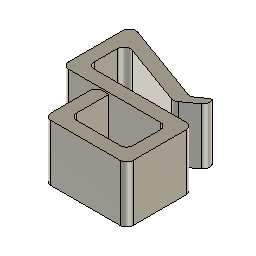
3-16ths wire clip (Autodesk Fusion 360 design; units mm, degrees)
Autodesk Fusion 360 part; units mm, degrees
sketch "Sketch1" plane through (0, 0, 0) normal (0, 0, 1) x (1, 0, 0)
  line L0 (0, 0) -> (-11.2763, 4.1042)
  line L1 (-11.2763, 4.1042) -> (-11.2763, -4.5808)
  line L2 (-11.2763, -4.5808) -> (1.7237, -4.5808)
  line L3 (1.7237, -4.5808) -> (1.7237, -9.5808)
  line L4 (1.7237, -9.5808) -> (-5.2763, -9.5808)
  line L5 (-6.8763, -11.1808) -> (3.3237, -11.1808)
  line L6 (3.3237, -11.1808) -> (3.3237, -2.9808)
  line L7 (3.3237, -2.9808) -> (-9.6763, -2.9808)
  line L8 (-9.6763, -2.9808) -> (-9.6763, 1.8192)
  line L9 (-9.6763, 1.8192) -> (-0.5472, -1.5035)
  line L10 (-9.6763, 1.8192) -> (-9.6763, -2.9808) construction
  line L11 (0, 0) -> (-0.5472, -1.5035)
  line L12 (-6.8763, -11.1808) -> (-6.8763, -4.7808)
  line L13 (-6.8763, -4.7808) -> (-5.2763, -4.7808)
  line L14 (-5.2763, -4.7808) -> (-5.2763, -9.5808)
  line L15 (-0.5472, -1.5035) -> (2.1518, 0.4308)
  line L16 (1.6257, 1.165) -> (0, 0)
  line L17 (2.1518, 0.4308) -> (1.6257, 1.165)
  dimension "d2" = 4.8
  dimension "d3" = 1.6
  dimension "d4" = 1.6
  dimension "d5" = 1.6
  dimension "d6" = 70
  dimension "d8" = 13
  dimension "d10" = 12
  dimension "d11" = 1.6
  dimension "d12" = 1.6
  dimension "d13" = 1.6
  dimension "d20" = 0.2
  dimension "d21" = 5
  dimension "d22" = 7
  dimension "d23" = 0.9033
  dimension "d24" = 2
  constraint perpendicular L2 L3
  constraint perpendicular L3 L4
  constraint perpendicular L4 L6
  constraint perpendicular L6 L7
  constraint parallel L1 L8
  constraint parallel L0 L9
  constraint coincident L7 L8.start
  constraint perpendicular L7 L10
  constraint perpendicular L9 L11
  constraint coincident L0.start L11.start
  constraint perpendicular L4 L12
  constraint perpendicular L4 L14
  constraint perpendicular L1 L2
  constraint parallel L15 L16
  constraint perpendicular L16 L17
  constraint horizontal L5
  measures "d2" distance of L8.end L7.end
  measures "d3" distance of L0 L9
  measures "d4" distance of L2 L7
  measures "d5" distance of L1 L8
  measures "d6" angle of L8 L9
  measures "d8" distance of L1.end L2.end
  measures "d10" distance of L0.start L0.end
  measures "d11" distance of L3 L6
  measures "d12" distance of L4 L5
  measures "d13" distance of L12 L14
  measures "d20" distance of L2 L13
  measures "d21" distance of L2.end L3.end
  measures "d22" distance of L3.end L4.end
  measures "d23" distance of L15 L16
  measures "d24" distance of L0.start L16.start
extrude "Extrude1" add sketch "Sketch1" along normal blind 7
fillet "Fillet1" radius 0.8 15 edges at (-11.2763, -4.5808, 3.5) (-6.8763, -11.1808, 3.5) (3.3237, -11.1808, 3.5) (3.3237, -2.9808, 3.5) (-9.6763, -2.9808, 3.5) (-5.2763, -9.5808, 3.5) (1.7237, -4.5808, 3.5) (1.7237, -9.5808, 3.5) (-11.2763, 4.1042, 3.5) (-9.6763, 1.8192, 3.5) (-0.5472, -1.5035, 3.5) (2.1518, 0.4308, 3.5) (1.6257, 1.165, 3.5) (0, 0, 3.5) (-6.8763, -4.7808, 3.5)
named bodies: "3-16 inch Wire Clip"
